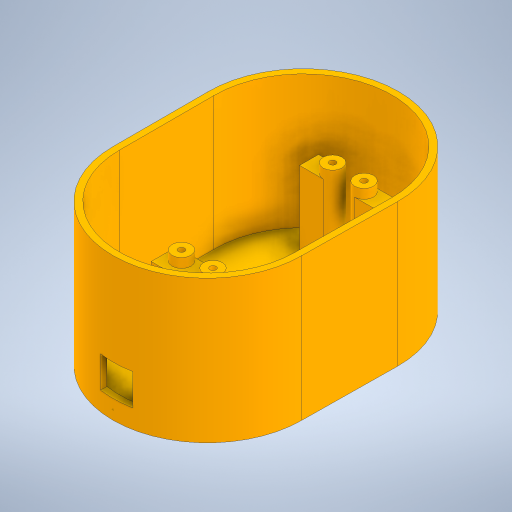
# Autodesk Inventor part: Base
Saved by Autodesk Inventor 2024 (Build 280153000, 153)
## iProperties
Created: 2024-04-28
Part Number: Base
Material: Generic
Document SubType Name: Modeling
Designer: samue
Density: 1 g/cm^3
Appearance: Default
Author: samue
## iProperties of the stored document Base_3DPrint.ipt
Created: 2024-04-28
Part Number: Base_3DPrint
Material: Generic
Document SubType Name: Modeling
Designer: samue
Density: 1 g/cm^3
Appearance: Default
Author: samue
Autodesk Inventor part; units mm, degrees
ref_plane "YZ Plane" through (0, 0, 0) normal (1, 0, 0) x (0, 1, 0)
ref_plane "XZ Plane" through (0, 0, 0) normal (0, 1, 0) x (-1, 0, 0)
ref_plane "XY Plane" through (0, 0, 0) normal (0, 0, 1) x (1, 0, 0)
sketch "Sketch10" plane through (0, 0, 0) normal (0, 1, 0) x (-1, 0, 0)
  arc A0 (30, 0) -> (-30, 0) centre (0, 0) ccw
  line L0 (30, 0) -> (30, -30)
  line L1 (-30, 0) -> (-30.34, -29.9981)
  arc A1 (-30.34, -29.9981) -> (30, -30) centre (-0.17, -30.34) ccw
  point P0 (0, 30)
  point P1 (0, 30)
  dimension "d39" = 60
  dimension "d40" = 30
  constraints: 5 point on circle, 4 end point, 2 centre point, 2 coincident, 2 tangent, 1 equal length, 1 vertical
  measures "d39" diameter of A0
  measures "d40" distance of L0.start L0.end
extrude "Extrusion10" add sketch "Sketch10" along normal blind 3
sketch "Sketch11" plane through (0, 3, 0) normal (0, 1, 0) x (1, 0, 0)
  arc A0 (-30, 0) -> (30, 0) centre (0, 0) ccw projected
  line L0 (-30, 30) -> (-30, 0) projected
  line L1 (30, 0) -> (30.34, 29.9981) projected
  arc A1 (30.34, 29.9981) -> (-30, 30) centre (0.17, 30.34) ccw projected
  line L2 (-30, 30) -> (-30, 0) projected
  arc A2 (-30, 0) -> (30, 0) centre (0, 0) ccw projected
  line L3 (-28, 30) -> (-28, 0)
  arc A3 (-28, 0) -> (28, 0) centre (0, 0) ccw
  arc A4 (28.3401, 30.0207) -> (-28, 30.0115) centre (0.17, 30.34) ccw
  line L4 (28.3401, 30.0207) -> (28, 0.0111)
  arc A5 (-28, 0) -> (28, 0.0111) centre (0, 0) ccw
  line L5 (-28, 0) -> (-28, 30.0115)
  point P0 (30, 0)
  point P1 (28, 0)
  dimension "d43" = 2
  dimension "d44" = 2
  constraints: 6 end point, 6 point on circle, 3 centre point, 4 other
  measures "d43" distance between parallel lines of L0 L3
  measures "d44" radial gap between concentric circles of A1 A4
extrude "Extrusion11" add sketch "Sketch11" along normal blind 42.3
sketch "Sketch12" plane through (0, 3, 0) normal (0, 1, 0) x (1, 0, 0)
  line L0 (-5, -3.2387) -> (5, -3.2387)
  line L1 (5, -3.2387) -> (5, 44.7613)
  line L2 (5, 44.7613) -> (-5, 44.7613)
  line L3 (-5, 44.7613) -> (-5, -3.2387)
  line L4 (-5, -3.2387) -> (5, 44.7613) construction
  line L5 (5, -3.2387) -> (-5, 44.7613) construction
  circle A0 centre (-5, -3.2387) radius 3
  circle A1 centre (-5, 44.7613) radius 3
  circle A2 centre (5, 44.7613) radius 3
  circle A3 centre (5, -3.2387) radius 3
  point P0 (0, 0)
  point P1 (0, 20.7613)
  dimension "d47" = 10
  dimension "d48" = 48
  dimension "d49" = 6
  dimension "d50" = 6
  dimension "d51" = 6
  dimension "d52" = 6
  constraints: 12 end point, 4 centre point, 4 coincident, 2 midpoint, 2 parallel, 1 horizontal, 1 perpendicular
  measures "d47" distance of L2.end L1.end
  measures "d48" distance of L1.end L0.end
  measures "d49" diameter of A0
  measures "d50" diameter of A1
  measures "d51" diameter of A2
  measures "d52" diameter of A3
extrude "Extrusion12" add sketch "Sketch12" along normal blind 28 contours L3 A0 L0 | L0 A0 L3 | A3 L1 L0 | L0 L1 A3 | A1 L2 L3 | L3 L2 A1 | A2 L2 L1 | L1 L2 A2
sketch "Sketch13" plane through (-5, 31, 3.2387) normal (0, 1, 0) x (1, 0, 0)
  circle A0 centre (0, 0) radius 3 projected
  circle A1 centre (10, 0) radius 3 projected
  circle A2 centre (0, 48) radius 3 projected
  circle A3 centre (10, 48) radius 3 projected
  circle A4 centre (0, 0) radius 1
  circle A5 centre (10, 0) radius 1
  circle A6 centre (0, 48) radius 1
  circle A7 centre (10, 48) radius 1
  point P0 (5, 3.2387)
  dimension "d55" = 2
  dimension "d56" = 2
  dimension "d57" = 2
  dimension "d58" = 2
  constraints: 4 centre point, 4 coincident
  measures "d55" diameter of A4
  measures "d56" diameter of A5
  measures "d57" diameter of A6
  measures "d58" diameter of A7
extrude "Extrusion13" cut sketch "Sketch13" against normal blind 14 contours A4 | A5 | A6 | A7
sketch "Sketch14" plane through (0, 3, 0) normal (0, 1, 0) x (1, 0, 0)
  line L0 (-9.6197, -0.2387) -> (10.3803, -0.2387)
  circle A0 centre (5, -3.2387) radius 3 projected
  circle A1 centre (-5, -3.2387) radius 3 projected
  line L1 (-9.6197, -0.2387) -> (-9.6197, -8.2414)
  line L2 (-9.6197, -8.2414) -> (10.3803, -8.2414)
  line L3 (10.3803, -8.2414) -> (10.3803, -0.2387)
  circle A2 centre (-5, 44.7613) radius 3 projected
  line L4 (-5, 47.7613) -> (-12.4823, 47.7613)
  line L5 (-12.4823, 47.7613) -> (-12.4823, 41.7613)
  line L6 (-12.4823, 41.7613) -> (-5, 41.7613)
  line L7 (0, 27.9217) -> (0, 57.8155) construction
  line L8 (5, 47.7613) -> (12.4823, 47.7613)
  line L9 (12.4823, 47.7613) -> (12.4823, 41.7613)
  line L10 (12.4823, 41.7613) -> (5, 41.7613)
  arc A3 (5, 41.7613) -> (5, 47.7613) centre (5, 44.7613) ccw
  point P0 (0, 0)
  point P1 (5, -0.2387)
  point P2 (-5, -0.2387)
  point P3 (5, 44.7613)
  dimension "d61" = 20
  constraints: 22 end point, 6 tangent, 5 symmetric about line, 4 point on circle, 3 vertical, 2 horizontal, 2 perpendicular, 1 centre point
  measures "d61" distance of L0.start L0.end
extrude "Extrusion14" add sketch "Sketch14" along normal blind 25 contours L0 L3 L2 L1
extrude "Extrusion15" add sketch "Sketch14" along normal blind 25 contours A2 L6 L5 L4 | L8 L9 L10 A3
sketch "Sketch15" plane through (0, 3, 0) normal (0, 1, 0) x (1, 0, 0)
  line L0 (-12.4823, 47.7613) -> (-5, 47.7613) projected
  line L1 (-12.4823, 47.7613) -> (-5, 47.7613)
  line L2 (-5, 47.7613) -> (-5, 50.6795)
  line L3 (-5, 50.6795) -> (-12.4823, 50.6795)
  line L4 (-12.4823, 50.6795) -> (-12.4823, 47.7613)
  point P0 (0, 0)
  constraints: 8 end point, 2 parallel, 1 horizontal, 1 perpendicular
extrude "Extrusion16" add sketch "Sketch15" along normal blind 3
mirror "Mirror2" about plane through (0, 0, 0) normal (1, 0, 0) of "Extrusion16"
sketch "Sketch16" plane through (0, 3, 0) normal (0, 1, 0) x (1, 0, 0)
  line L0 (10.3803, -8.2414) -> (-9.6197, -8.2414) projected
  line L1 (-9.6197, -8.2414) -> (10.3803, -8.2414)
  line L2 (10.3803, -8.2414) -> (10.3803, -10.45)
  line L3 (10.3803, -10.45) -> (-9.6197, -10.45)
  line L4 (-9.6197, -10.45) -> (-9.6197, -8.2414)
  point P0 (0, 0)
  constraints: 8 end point, 2 parallel, 1 horizontal, 1 perpendicular
extrude "Extrusion17" add sketch "Sketch16" along normal blind 3
sketch "Sketch17" plane through (-9.6197, 28, 8.2414) normal (0, 0, 1) x (1, 0, 0)
  line L0 (0, -22) -> (20, -22) projected
  line L1 (5.3464, -22) -> (15.3464, -22)
  line L2 (15.3464, -22) -> (15.3464, -12)
  line L3 (15.3464, -12) -> (5.3464, -12)
  line L4 (5.3464, -12) -> (5.3464, -22)
  point P0 (9.6197, -28)
  dimension "d70" = 10
  dimension "d71" = 10
  constraints: 8 end point, 2 parallel, 1 horizontal, 1 perpendicular, 1 point on line
  measures "d70" distance of L3.end L2.end
  measures "d71" distance of L2.end L1.end
extrude "Extrusion18" cut sketch "Sketch17" along normal blind 34.75
body "Solid2"
